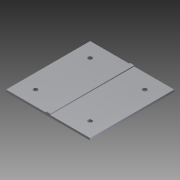
# Autodesk Inventor part: base
Saved by Autodesk Inventor 2011 (Build 150239000, 239)
## iProperties
Created: 2011-07-09
Part Number: base
Document SubType Name: Modeling
Designer: adowning
Density: 1 g/cm^3
Author: adowning
Autodesk Inventor part; units mm, degrees
ref_plane "YZ Plane" through (0, 0, 0) normal (1, 0, 0) x (0, 1, 0)
ref_plane "XZ Plane" through (0, 0, 0) normal (0, 1, 0) x (-1, 0, 0)
ref_plane "XY Plane" through (0, 0, 0) normal (0, 0, 1) x (1, 0, 0)
sketch "Sketch1" plane through (0, 0, 0) normal (0, 0, 1) x (1, 0, 0)
  point P0 (0, 0)
sketch "Sketch2" plane through (0, 0, 0) normal (0, 1, 0) x (-1, 0, 0)
  line L0 (205.3066, 309.3165) -> (-302.6934, 309.3165)
  line L1 (-302.6934, 309.3165) -> (-302.6934, -198.6835)
  line L2 (-302.6934, -198.6835) -> (205.3066, -198.6835)
  line L3 (205.3066, -198.6835) -> (205.3066, 309.3165)
  point P0 (0, 0)
  dimension "d0" = 508
  dimension "d1" = 508
  constraints: 8 end point, 2 parallel, 1 horizontal, 1 perpendicular
  measures "d0" distance of L2.end L1.end
  measures "d1" distance of L1.end L0.end
extrude "Extrusion1" add sketch "Sketch2" along normal blind 12.7
sketch "Sketch3" plane through (0, 12.7, 0) normal (0, 1, 0) x (1, 0, 0)
  line L0 (-205.3066, -309.3165) -> (-116.4066, -309.3165)
  line L1 (-116.4066, -309.3165) -> (-116.4066, -220.4165)
  line L2 (-116.4066, -220.4165) -> (-205.3066, -220.4165)
  line L3 (-205.3066, -220.4165) -> (-205.3066, -309.3165)
  line L4 (-205.3066, 198.6835) -> (-116.4066, 198.6835)
  line L5 (-116.4066, 198.6835) -> (-116.4066, 109.7835)
  line L6 (-116.4066, 109.7835) -> (-205.3066, 109.7835)
  line L7 (-205.3066, 109.7835) -> (-205.3066, 198.6835)
  line L8 (302.6934, 198.6835) -> (213.7934, 198.6835)
  line L9 (213.7934, 198.6835) -> (213.7934, 109.7835)
  line L10 (213.7934, 109.7835) -> (302.6934, 109.7835)
  line L11 (302.6934, 109.7835) -> (302.6934, 198.6835)
  line L12 (302.6934, -309.3165) -> (213.7934, -309.3165)
  line L13 (213.7934, -309.3165) -> (213.7934, -220.4165)
  line L14 (213.7934, -220.4165) -> (302.6934, -220.4165)
  line L15 (302.6934, -220.4165) -> (302.6934, -309.3165)
  circle A0 centre (-116.4066, -220.4165) radius 12.7
  circle A1 centre (-116.4066, 109.7835) radius 12.7
  circle A2 centre (213.7934, 109.7835) radius 12.7
  circle A3 centre (213.7934, -220.4165) radius 12.7
  point P0 (0, 0)
  dimension "d4" = 88.9
  dimension "d5" = 88.9
  dimension "d6" = 88.9
  dimension "d7" = 88.9
  dimension "d8" = 88.9
  dimension "d9" = 88.9
  dimension "d10" = 88.9
  dimension "d11" = 88.9
  dimension "d12" = 25.4
  dimension "d13" = 25.4
  dimension "d14" = 25.4
  dimension "d15" = 25.4
  constraints: 32 end point, 8 parallel, 4 centre point, 4 coincident, 4 horizontal, 4 perpendicular
  measures "d4" distance of L2.end L1.end
  measures "d5" distance of L1.end L0.end
  measures "d6" distance of L5.end L6.end
  measures "d7" distance of L4.end L5.end
  measures "d8" distance of L10.end L9.end
  measures "d9" distance of L9.end L8.end
  measures "d10" distance of L13.end L14.end
  measures "d11" distance of L12.end L13.end
  measures "d12" diameter of A0
  measures "d13" diameter of A1
  measures "d14" diameter of A2
  measures "d15" diameter of A3
extrude "Extrusion2" cut sketch "Sketch3" against normal blind 12.7 contours A0 L2 L1 | L1 L2 A0 | A1 L6 L5 | L5 L6 A1 | A2 L10 L9 | L9 L10 A2 | A3 L14 L13 | L13 L14 A3
sketch "Sketch4" plane through (0, 12.7, 0) normal (0, 1, 0) x (1, 0, 0)
  line L0 (302.6934, -309.3165) -> (-205.3066, -309.3165) projected
  line L1 (-205.3066, 198.6835) -> (302.6934, 198.6835) projected
  line L2 (302.6934, 198.6835) -> (48.6934, 198.6835)
  line L3 (48.6934, 198.6835) -> (74.0934, 198.6835)
  line L4 (74.0934, 198.6835) -> (61.3934, 198.6835)
  line L5 (61.3934, 198.6835) -> (35.9934, 198.6835)
  line L6 (35.9934, 198.6835) -> (35.9934, -309.3165)
  line L7 (35.9934, -309.3165) -> (61.3934, -309.3165)
  line L8 (61.3934, -309.3165) -> (61.3934, 198.6835)
  line L9 (61.3934, 198.6835) -> (35.9934, 198.6835)
  line L10 (35.9934, 198.6835) -> (35.9934, -309.3165)
  point P0 (0, 0)
  dimension "d18" = 254
  dimension "d19" = 25.4
  dimension "d20" = 12.7
  dimension "d21" = 25.4
  constraints: 18 end point, 3 point on line, 2 midpoint, 2 parallel, 2 perpendicular, 1 horizontal
  measures "d18" distance of L1.end L2.end
  measures "d19" distance of L2.end L3.end
  measures "d20" distance of L3.end L4.end
  measures "d21" distance of L4.end L5.end
extrude "Extrusion3" add sketch "Sketch4" along normal blind 6.35
body "Solid1"
